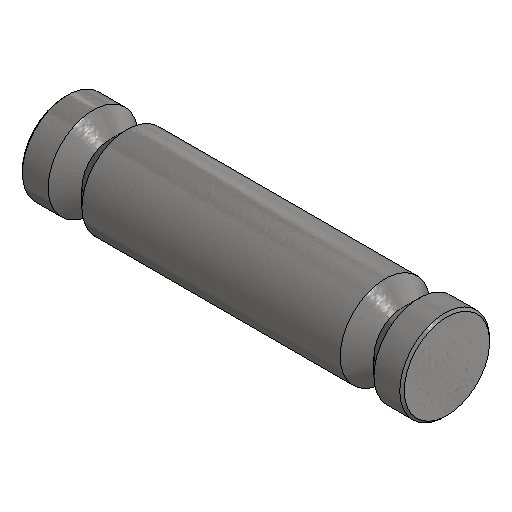
# Autodesk Inventor part: TL20240701-10100AT-002
Saved by Autodesk Inventor 2022.5 (Build 265521000, 521)
## iProperties
Category: ANTI BACK ASSY
Company: 현대트랜시스(대유)
RuleStatus: InUse
Part Number: TL20240701-10100AT-002
Project: SW-PJT
Checked By: 김형민
Engr Approved By: 김시현
User Status: 1 x78
Material: S45C
Description: 0
Document SubType Name: Modeling
Mfg Approved By: 호상태
Designer: USER106
Stock Number: 002
Density: 7.87 g/cm^3
Appearance: Plating Zinc White
Detail Description: Processed products
Title: SHAFT
Subject: SW차종 시트조립라인
Author: USER106
Revision Number: A
Autodesk Inventor part; units mm, degrees
ref_plane "YZ Plane" through (0, 0, 0) normal (1, 0, 0) x (0, 1, 0)
ref_plane "XZ Plane" through (0, 0, 0) normal (0, 1, 0) x (-1, 0, 0)
ref_plane "XY Plane" through (0, 0, 0) normal (0, 0, 1) x (1, 0, 0)
sketch "Sketch2" plane through (0, 0, 0) normal (0, 0, 1) x (1, 0, 0)
  line L0 (-17, 0) -> (17, 0)
  line L1 (-17, 0) -> (-17, -4)
  line L2 (-17, -4) -> (-14.5, -4)
  line L3 (-14.5, -4) -> (-13, -2.5)
  line L4 (-13, -2.5) -> (-11.5, -4)
  line L5 (-11.5, -4) -> (0, -4)
  line L6 (0, 0) -> (0, -4) construction
  line L7 (-13, -2.5) -> (-13, 0) construction
  line L8 (17, 0) -> (17, -4)
  line L9 (17, -4) -> (14.5, -4)
  line L10 (14.5, -4) -> (13, -2.5)
  line L11 (13, -2.5) -> (11.5, -4)
  line L12 (11.5, -4) -> (0, -4)
  dimension "d1" = 34
  dimension "d2" = 135
  dimension "d3" = 4
  dimension "d4" = 8
  dimension "d5" = 3
  constraints: 26 end point, 4 symmetric about line, 3 perpendicular, 2 collinear, 2 vertical, 1 coincident, 1 horizontal, 1 midpoint, 1 point on line
  measures "d1" distance of L0.start L0.end
  measures "d2" angle of L2 L3
  measures "d3" distance between parallel lines of L7 L1
  measures "d4" diameter of L2 L0
  measures "d5" distance of L2.end L4.end
revolve "Revolution1" add sketch "Sketch2" angle 360 about axis through (-17, 0, 0) along (1, 0, 0)
chamfer "Chamfer1" distance 0.2 angle 45 2 edges at (-17, 4, 0) (17, 4, 0)
body "Solid1"
